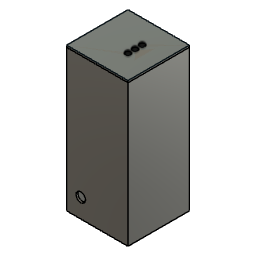
PF last (Autodesk Fusion 360 design; units mm, degrees)
Autodesk Fusion 360 part; units mm, degrees
sketch "Boceto2" plane through (0, 0, 0) normal (0, 1, 0) x (1, 0, 0)
  line L0 (0, 0) -> (-65, 0)
  line L1 (-65, 0) -> (-65, 65)
  line L2 (-65, 65) -> (0, 65)
  line L3 (0, 65) -> (0, 0)
  dimension "d3" = 65
  dimension "d4" = 65
  constraint horizontal L0
  constraint vertical L1
  constraint horizontal L2
  constraint vertical L3
  constraint coincident L0.start L3.end
  measures "d3" distance of L0.start L2.end
  measures "d4" distance of L0.start L0.end
extrude "Extruir3" add sketch "Boceto2" along normal blind 150 makes body 1
sketch "Boceto4" plane through (0, 150, 0) normal (0, 1, 0) x (-1, 0, 0)
  line L0 (0, -65) -> (65, -65)
  line L1 (65, -65) -> (65, 0)
  line L2 (65, 0) -> (0, 0)
  line L3 (0, 0) -> (0, -65)
  line L4 (5, -2) -> (63, -2)
  line L5 (63, -2) -> (63, -63)
  line L6 (63, -63) -> (5, -63)
  line L7 (5, -63) -> (5, -2)
  dimension "d13" = 5
  dimension "d14" = 2
  dimension "d15" = 2
  dimension "d16" = 2
  constraint horizontal L4
  constraint vertical L5
  constraint horizontal L6
  constraint vertical L7
  measures "d13" distance of L3 L7
  measures "d14" distance of L0 L6
  measures "d15" distance of L1 L5
  measures "d16" distance of L2 L4
extrude "Extruir5" cut sketch "Boceto4" against normal blind 149 contours L4 L5 L6 L7 bodies 1
sketch "Boceto5" plane through (0, 150, 0) normal (0, 1, 0) x (-1, 0, 0)
  line L0 (63, -2) -> (63, -63)
  line L1 (63, -63) -> (5, -63)
  line L2 (5, -63) -> (5, -2)
  line L3 (5, -2) -> (63, -2)
  line L4 (0, -65) -> (65, -65)
  line L5 (65, -65) -> (65, 0)
  line L6 (65, 0) -> (0, 0)
  line L7 (0, 0) -> (0, -65)
  line L8 (0, 0) -> (65, 0)
  line L9 (65, 0) -> (65, -65)
  line L10 (65, -65) -> (0, -65)
  line L11 (0, -65) -> (0, 0)
  constraint horizontal L8
  constraint vertical L9
  constraint horizontal L10
  constraint vertical L11
  constraint coincident L4.end L5.start
  constraint coincident L6.end L7.start
extrude "Extruir6" add sketch "Boceto5" along normal blind 2 separate body contours L0 L1 L2 L3 | L4 L5 L6 L7 L8 L9 L10 L11 makes body 2
sketch "Boceto6" plane through (0, 150, 0) normal (0, -1, 0) x (1, 0, 0)
  line L0 (-65, -65) -> (0, -65)
  line L1 (0, -65) -> (0, 0)
  line L2 (0, 0) -> (-65, 0)
  line L3 (-65, 0) -> (-65, -65)
  line L4 (-5.5, -62.5) -> (-62.5, -62.5)
  line L5 (-62.5, -62.5) -> (-62.5, -2.5)
  line L6 (-62.5, -2.5) -> (-5.5, -2.5)
  line L7 (-5.5, -2.5) -> (-5.5, -62.5)
  dimension "d21" = 5.5
  dimension "d22" = 2.5
  dimension "d23" = 2.5
  dimension "d24" = 2.5
  constraint horizontal L4
  constraint vertical L5
  constraint horizontal L6
  constraint vertical L7
  measures "d21" distance of L1 L7
  measures "d22" distance of L2 L6
  measures "d23" distance of L3 L5
  measures "d24" distance of L0 L4
extrude "Extruir7" add sketch "Boceto6" along normal blind 2 contours L4 L5 L6 L7 bodies 2
sketch "Boceto7" plane through (0, 0, 0) normal (0, 0, 1) x (1, 0, 0)
  line L0 (-65, 0) -> (0, 0)
  line L1 (0, 0) -> (0, 150)
  line L2 (0, 150) -> (-65, 150)
  line L3 (-65, 150) -> (-65, 0)
  circle A0 centre (-50, 20) radius 5
  dimension "d27" = 10
  measures "d27" diameter of A0
extrude "Extruir8" cut sketch "Boceto7" against normal up to surface (2 mm away) contours A0 bodies 1
sketch "Boceto8" plane through (0, 152, 0) normal (0, 1, 0) x (-1, 0, 0)
  line L0 (0, -65) -> (65, -65)
  line L1 (65, -65) -> (65, 0)
  line L2 (65, 0) -> (0, 0)
  line L3 (0, 0) -> (0, -65)
  circle A0 centre (25, -25) radius 2.5
  circle A1 centre (25, -32.5) radius 2.5
  circle A2 centre (25, -40) radius 2.5
  dimension "d31" = 5
  dimension "d32" = 5
  dimension "d33" = 5
  dimension "d34" = 25
  dimension "d35" = 25
  dimension "d36" = 25
  dimension "d37" = 25
  dimension "d38" = 32.5
  dimension "d39" = 25
  measures "d31" diameter of A0
  measures "d32" diameter of A1
  measures "d33" diameter of A2
  measures "d34" distance of L3 A2.centre
  measures "d35" distance of L3 A1.centre
  measures "d36" distance of L3 A0.centre
  measures "d37" distance of L2 A0.centre
  measures "d38" distance of L2 A1.centre
  measures "d39" distance of L0 A2.centre
named bodies: "caja", "tapiña"
